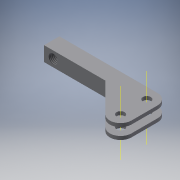
# Autodesk Inventor part: newfrontpart
Saved by Autodesk Inventor 2018 (Build 220112000, 112)
## iProperties
Created: 2018-12-03
Part Number: newfrontpart
Material: Generic
Document SubType Name: Modeling
Designer: Jerry
Density: 1 g/cm^3
Appearance: Default
Author: Jerry
Autodesk Inventor part; units mm, degrees
ref_plane "YZ Plane" through (0, 0, 0) normal (1, 0, 0) x (0, 1, 0)
ref_plane "XZ Plane" through (0, 0, 0) normal (0, 1, 0) x (-1, 0, 0)
ref_plane "XY Plane" through (0, 0, 0) normal (0, 0, 1) x (1, 0, 0)
sketch "Sketch1" plane through (0, 0, 0) normal (0, 0, 1) x (1, 0, 0)
  line L0 (0, 0) -> (64, 0)
  arc A0 (71, -7) -> (64, 0) centre (64, -7) ccw
  line L1 (64, 0) -> (64, -7) construction
  line L2 (71, -7) -> (64, -7) construction
  line L3 (0, 0) -> (0, -10)
  line L4 (0, -10) -> (40, -10)
  line L5 (40, -10) -> (59.0503, -29.0503)
  line L6 (71, -24.1005) -> (71, -7)
  arc A1 (59.0503, -29.0503) -> (71, -24.1005) centre (64, -24.1005) ccw
  line L7 (51, 0) -> (51, -21)
  dimension "d0" = 64
  dimension "d1" = 7
  dimension "d2" = 90
  dimension "d3" = 10
  dimension "d4" = 40
  dimension "d5" = 90
  dimension "d6" = 135
  dimension "d7" = 7
  dimension "d8" = 20
  constraints: 16 end point, 4 point on circle, 3 tangent, 2 centre point, 2 perpendicular, 2 point on line, 1 horizontal, 1 parallel, 1 vertical
  measures "d0" distance of L0.start L0.end
  measures "d1" radius of A0
  measures "d2" angle of L2 L1
  measures "d3" distance of L0.start L3.end
  measures "d4" distance of L3.end L4.end
  measures "d5" angle of L4 L3
  measures "d6" angle of L4 L5
  measures "d7" radius of A1
  measures "d8" distance between parallel lines of L6 L7
extrude "Extrusion1" add sketch "Sketch1" along normal mid plane 9.525
extrude "Extrusion2" cut sketch "Sketch1" along normal mid plane 5 contours L0 A0 L6 A1 L5 L7
hole "Hole1" at (64, -7, 0) at (64, -24.1005, 0) direction (0, 0, -1) diameter 5.159 end through all both
sketch "Sketch2" plane through (0, 0, -4.7625) normal (0, 1, 0) x (1, 0, 0)
  line L0 (64, -7.2625) -> (51, -7.2625) projected
  line L1 (51, -7.2625) -> (51, -2.2625) projected
  line L2 (51, -2.2625) -> (64, -2.2625) projected
  line L3 (64, -2.2625) -> (64, 0) projected
  line L4 (0, 0) -> (64, 0) projected
  line L5 (0, -9.525) -> (0, 0) projected
  line L6 (64, -9.525) -> (0, -9.525) projected
  line L7 (64, -9.525) -> (64, -7.2625) projected
  point P0 (0, -4.7625)
  point P1 (6, -4.7625)
  point P2 (0, -4.7625)
  dimension "d20" = 6
  constraints: 1 horizontal alignment, 1 midpoint
  measures "d20" distance from line of L5 point (6, -4.763)
hole "Hole2" at (6, 0, 0) direction (0, -1, 0) diameter 6 end through all
thread "Thread1" size "M6x1" class "6H" standard "ANSI Metric M Profile" full length
equation "\"d7\" = d1"
body "Solid1"
